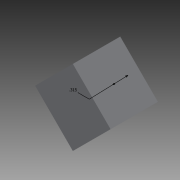
# Autodesk Inventor part: Driver Shaft
Saved by Autodesk Inventor 2018 (Build 220112000, 112)
## iProperties
Created: 2018-01-21
Part Number: Driver Shaft
Material: Generic
Document SubType Name: Modeling
Designer: Rus
Density: 1 g/cm^3
Appearance: Default
Author: Rus
Autodesk Inventor part; units mm, degrees
ref_plane "YZ Plane" through (0, 0, 0) normal (1, 0, 0) x (0, 1, 0)
ref_plane "XZ Plane" through (0, 0, 0) normal (0, 1, 0) x (-1, 0, 0)
ref_plane "XY Plane" through (0, 0, 0) normal (0, 0, 1) x (1, 0, 0)
sketch "Sketch1" plane through (0, 0, 0) normal (0, 0, 1) x (1, 0, 0)
  line L0 (13.4704, 0) -> (0, -13.4704)
  line L1 (0, -13.4704) -> (-13.4704, 0)
  line L2 (-13.4704, 0) -> (0, 13.4704)
  line L3 (0, 13.4704) -> (13.4704, 0)
  line L4 (0, 0) -> (0, 13.4704) construction
  dimension "d0" = 19.05
  constraints: 10 end point, 1 coincident, 1 vertical, 9 other
  measures "d0" distance of L2.end L0.start
extrude "Extrusion1" add sketch "Sketch1" against normal blind 16.9333
sketch "Sketch2" plane through (0, 0, -16.9333) normal (0, 0, -1) x (-1, 0, 0)
  circle A0 centre (0, 0) radius 4
  dimension "d3" = 8
  constraints: 1 centre point, 1 coincident
  measures "d3" diameter of A0
body "Solid1"
